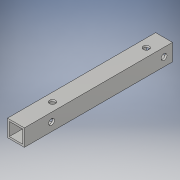
# Autodesk Inventor part: ハンド_角柱2
Saved by Autodesk Inventor 2019.4 (Build 234330000, 330)
## iProperties
Created: 2021-12-06
Part Number: ハンド_角柱2
Material: アルミニウム 6061
Document SubType Name: Modeling
Designer: 堀川皓史
Density: 2.7 g/cm^3
Appearance: アルミニウム - フラット
Author: 堀川皓史
Autodesk Inventor part; units mm, degrees
ref_plane "YZ Plane" through (0, 0, 0) normal (1, 0, 0) x (0, 1, 0)
ref_plane "XZ Plane" through (0, 0, 0) normal (0, 1, 0) x (-1, 0, 0)
ref_plane "XY Plane" through (0, 0, 0) normal (0, 0, 1) x (1, 0, 0)
sketch "スケッチ1" plane through (0, 0, 0) normal (0, 0, 1) x (1, 0, 0)
  line L0 (4.5, 4.5) -> (-4.5, 4.5)
  line L1 (-4.5, 4.5) -> (-4.5, -4.5)
  line L2 (-4.5, -4.5) -> (4.5, -4.5)
  line L3 (4.5, -4.5) -> (4.5, 4.5)
  line L4 (4.5, 4.5) -> (-4.5, -4.5) construction
  line L5 (-4.5, 4.5) -> (4.5, -4.5) construction
  line L6 (-3.5, 3.5) -> (3.5, 3.5)
  line L7 (3.5, 3.5) -> (3.5, -3.5)
  line L8 (3.5, -3.5) -> (-3.5, -3.5)
  line L9 (-3.5, -3.5) -> (-3.5, 3.5)
  point P0 (0, 0)
  dimension "d0" = 9
  dimension "d1" = 9
  dimension "d2" = 1
  constraints: 20 end point, 4 parallel, 2 midpoint, 2 perpendicular, 1 horizontal, 3 other
  measures "d0" distance of L2.end L1.end
  measures "d1" distance of L1.end L0.end
  measures "d2" distance between parallel lines of L0 L6
extrude "押し出し1" add sketch "スケッチ1" along normal blind 79
sketch "スケッチ2" plane through (4.5, -4.5, 0) normal (1, 0, 0) x (0, 0, -1)
  circle A0 centre (-4.5, 4.5) radius 1.6
  circle A1 centre (-64.5, 4.5) radius 1.6
  line L0 (0, 0) -> (0, 9) projected
  point P0 (0, 4.5)
  point P1 (0, 4.5)
  dimension "d5" = 3.2
  dimension "d6" = 3.2
  dimension "d7" = 4.5
  dimension "d8" = 60
  constraints: 2 centre point, 2 horizontal alignment, 1 midpoint
  measures "d5" diameter of A0
  measures "d6" diameter of A1
  measures "d7" distance of point (0, 4.5) A0.centre
  measures "d8" distance of A0.centre A1.centre
extrude "押し出し2" cut sketch "スケッチ2" against normal through all
sketch "スケッチ3" plane through (-4.5, 4.5, 0) normal (0, 1, 0) x (1, 0, 0)
  circle A0 centre (4.5, -9.5) radius 1.6
  circle A1 centre (4.5, -59.5) radius 1.6
  line L0 (9, 0) -> (0, 0) projected
  point P0 (4.5, 0)
  point P1 (4.5, 0)
  dimension "d11" = 3.2
  dimension "d12" = 3.2
  dimension "d13" = 50
  dimension "d14" = 9.5
  constraints: 2 centre point, 2 vertical alignment, 1 midpoint
  measures "d11" diameter of A0
  measures "d12" diameter of A1
  measures "d13" distance of A0.centre A1.centre
  measures "d14" distance of point (4.5, 0) A0.centre
extrude "押し出し3" cut sketch "スケッチ3" against normal through all
